box_lid (Autodesk Fusion 360 design; units mm, degrees)
Autodesk Fusion 360 part; units mm, degrees
sketch "Sketch1" plane through (0, 0, 0) normal (0, 1, 0) x (1, 0, 0)
  line L0 (0, 0) -> (33.5, 0)
  line L1 (27.75, -33) -> (27.75, -45)
  line L2 (27.75, -45) -> (5.75, -45)
  line L3 (5.75, -45) -> (5.75, -33)
  line L4 (33.5, -33) -> (27.75, -33)
  line L5 (5.75, -33) -> (0, -33)
  line L6 (-2, -35) -> (-2, 2)
  line L7 (-2, 2) -> (35.5, 2)
  line L8 (35.5, 2) -> (35.5, -35)
  line L9 (35.5, -35) -> (29.75, -35)
  line L10 (29.75, -35) -> (29.75, -47)
  line L11 (29.75, -47) -> (3.75, -47)
  line L12 (3.75, -47) -> (3.75, -35)
  line L13 (3.75, -35) -> (-2, -35)
  line L14 (33.5, -33) -> (33.5, -28)
  line L15 (33.5, -28) -> (34.5, -28)
  line L16 (34.5, -28) -> (34.5, -5)
  line L17 (34.5, -5) -> (33.5, -5)
  line L18 (33.5, -5) -> (33.5, 0)
  line L19 (0, -33) -> (0, -28)
  line L20 (0, -28) -> (-1, -28)
  line L21 (-1, -28) -> (-1, -5)
  line L22 (-1, -5) -> (0, -5)
  line L23 (0, -5) -> (0, 0)
  line L24 (0, -28) -> (0, -5)
  line L25 (33.5, -28) -> (33.5, -5)
  dimension "d1" = 33.5
  dimension "d3" = 33
  dimension "d4" = 22
  dimension "d5" = 5.75
  dimension "d6" = 5.75
  dimension "d7" = 12
  dimension "d8" = 2
  dimension "d9" = 2
  dimension "d10" = 2
  dimension "d12" = 2
  dimension "d14" = 2
  dimension "d15" = 2
  dimension "d39" = 5
  dimension "d40" = 5
  dimension "d41" = 5
  dimension "d42" = 5
  dimension "d43" = 1
  dimension "d44" = 1
  dimension "d45" = 33
  dimension "d46" = 35.5
  constraint horizontal L0
  constraint horizontal L4
  constraint vertical L1
  constraint horizontal L2
  constraint vertical L3
  constraint coincident L3.end L4
  constraint collinear L4 L5
  constraint coincident L0.start L23.end
  constraint perpendicular L6 L7
  constraint perpendicular L7 L8
  constraint perpendicular L8 L9
  constraint perpendicular L2 L10
  constraint perpendicular L10 L11
  constraint perpendicular L11 L12
  constraint perpendicular L6 L13
  constraint perpendicular L4 L14
  constraint perpendicular L8 L15
  constraint perpendicular L4 L16
  constraint perpendicular L16 L17
  constraint perpendicular L0 L18
  constraint perpendicular L5 L19
  constraint perpendicular L19 L20
  constraint perpendicular L5 L21
  constraint perpendicular L21 L22
  constraint perpendicular L0 L23
  constraint perpendicular L17 L25
  measures "d1" distance of L0.start L0.end
  measures "d3" distance of L0.start L5.end
  measures "d4" distance of L1.end L2.end
  measures "d5" distance of L4.start L1.start
  measures "d6" distance of L5.end L3.end
  measures "d7" distance of L3.end L2.end
  measures "d9" distance of L1 L10
  measures "d10" distance of L4 L9
  measures "d12" distance of L0 L7
  measures "d14" distance of L5 L13
  measures "d15" distance of L3 L12
  measures "d39" distance of L4.start L14.end
  measures "d40" distance of L0.end L17.end
  measures "d41" distance of L0.start L22.end
  measures "d42" distance of L5.end L19.end
  measures "d43" distance of L6 L21
  measures "d44" distance of L8 L16
  measures "d45" distance of L0 L5
  measures "d46" distance of L16 L21
extrude "Extrude1" add sketch "Sketch1" against normal blind 2 contours L0 L1 L2 L3 L4 L5 L14 L18 L19 L23 L24 L25 | L20 L21 L22 L24 | L15 L16 L17 L25 | L6 L7 L8 L9 L10 L11 L12 L13
extrude "Extrude3" add sketch "Sketch1" along normal blind 10 contours L20 L21 L22 L24 | L15 L16 L17 L25
fillet "Fillet2" radius 2 8 edges at (3.75, -1, 47) (29.75, -1, 47) (29.75, -1, 35) (35.5, -1, 35) (35.5, -1, -2) (-2, -1, -2) (-2, -1, 35) (3.75, -1, 35)
chamfer "Chamfer2" distance 1 angle 45 16 edges at (4.3358, -2, 46.4142) (3.75, -2, 41) (3.1642, -2, 35.5858) (0.875, -2, 35) (-1.4142, -2, 34.4142) (-2, -2, 16.5) (-1.4142, -2, -1.4142) (16.75, -2, -2) (34.9142, -2, -1.4142) (35.5, -2, 16.5) (34.9142, -2, 34.4142) (32.625, -2, 35) (30.3358, -2, 35.5858) (29.75, -2, 41) (29.1642, -2, 46.4142) (16.75, -2, 47)
extrude "Extrude2" [suppressed]
hole "Hole1" [suppressed]
sketch "Sketch2" plane through (0, 0, 47) normal (0, 0, 1) x (-1, 0, 0)
  line L0 (-3.75, -23) -> (-3.75, 2)
  line L1 (-3.75, 2) -> (-29.75, 2)
  line L2 (-29.75, 2) -> (-29.75, -23)
  line L3 (-29.75, -23) -> (-3.75, -23)
  circle A0 centre (-16.25, -6) radius 1.55
  circle A1 centre (-14.8465, -7.8641) radius 1.55
  dimension "d23" = 3.1
  dimension "d24" = 13.5
  dimension "d25" = 17
  measures "d23" diameter of A0
  measures "d24" distance of L2 A0.centre
  measures "d25" distance of L3 A0.centre
hole "Hole2" [suppressed]
fillet "Fillet1" [suppressed]
